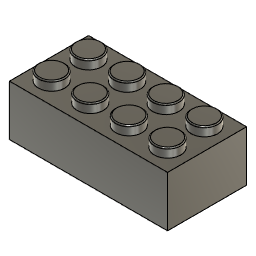
lago v2 (Autodesk Fusion 360 design; units mm, degrees)
Autodesk Fusion 360 part; units mm, degrees
note: some values were not read from the file. Set by a fixed rule: which face or edge a step refers to.
sketch "Sketch1" plane through (0, 0, 0) normal (0, 0, 1) x (1, 0, 0) in component "lago"
  line L0 (0, 0) -> (30, 0)
  line L1 (30, 0) -> (30, 15)
  line L2 (30, 15) -> (0, 15)
  line L3 (0, 15) -> (0, 0)
  constraint horizontal L0
  constraint vertical L1
  constraint horizontal L2
  constraint vertical L3
  constraint coincident L0.start L3.end
extrude "Extrude1" add sketch "Sketch1" along normal blind 9.6 in component "lago"
sketch "Sketch2" plane through (0, 0, 9.6) normal (0, 0, 1) x (-1, 0, 0) in component "lago"
  line L0 (0, -15) -> (0, 0)
  line L1 (0, 0) -> (-30, 0)
  line L2 (-30, 0) -> (-30, -15)
  line L3 (-30, -15) -> (0, -15)
  circle A0 centre (-3.9, -11.1) radius 2.5
  dimension "d3" = 5
  dimension "d4" = 3.9
  dimension "d5" = 3.9
  measures "d3" diameter of A0
  measures "d4" distance of L3 A0.centre
  measures "d5" distance of L0 A0.centre
extrude "Extrude2" add sketch "Sketch2" along normal blind 1.7 contours A0 in component "lago"
pattern_linear "R-Pattern1" count 4 spacing 7.3333 along (1, 0, 0) count 2 spacing 7 along (0, -1, 0) of "Extrude2" in component "lago"
shell "Shell1" thickness 1.3 removed faces 1 at (10, 5, 0) in component "lago"
sketch "Sketch3" plane through (0, 0, 8.3) normal (0, 0, -1) x (1, 0, 0) in component "lago"
  circle A0 centre (25.9, -4.1) radius 1.2
  circle A1 centre (18.5667, -4.1) radius 1.2
  circle A2 centre (11.2333, -4.1) radius 1.2
  circle A3 centre (3.9, -4.1) radius 1.2
  circle A4 centre (25.9, -11.1) radius 1.2
  circle A5 centre (18.5667, -11.1) radius 1.2
  circle A6 centre (11.2333, -11.1) radius 1.2
  circle A7 centre (3.9, -11.1) radius 1.2
  line L0 (1.3, -1.3) -> (1.3, -13.7)
  line L1 (1.3, -13.7) -> (28.7, -13.7)
  line L2 (28.7, -13.7) -> (28.7, -1.3)
  line L3 (28.7, -1.3) -> (1.3, -1.3)
  line L4 (11.2333, -4.1) -> (3.9, -11.1) construction
  circle A8 centre (7.5667, -7.6) radius 2.3581
  circle A9 centre (7.5667, -7.6) radius 3.3581
  dimension "d13" = 1
  constraint coincident A2.centre L4.start
  constraint coincident A7.centre L4.end
  constraint midpoint L4 A8.centre
extrude "Extrude3" add sketch "Sketch3" along normal blind 8 contours A9 in component "lago"
pattern_linear "R-Pattern2" count 3 spacing 7.5 along (1, 0, 0) of "Extrude3" in component "lago"
fillet "Fillet1" radius 0.2 8 edges at (28.2308, 12.004, 11.3) (28.2308, 5.004, 11.3) (20.8975, 5.004, 11.3) (20.8975, 12.004, 11.3) (13.5642, 5.004, 11.3) (13.5642, 12.004, 11.3) (6.2308, 12.004, 11.3) (6.2308, 5.004, 11.3) in component "lago"
fillet "Fillet2" radius 0.02 3 edges at (19.4358, 8.8143, 0.3) (11.9358, 8.8143, 0.3) (4.4358, 8.8143, 0.3) in component "lago"
fillet "Fillet3" radius 0.02 2 edges at (11.9358, 6.3857, 8.3) (4.4358, 6.3857, 8.3) in component "lago"
fillet "Fillet4" radius 0.2 1 edges at (19.4358, 6.3857, 8.3) in component "lago"
fillet "Fillet5" radius 0.2 13 faces at (10.5569, 7.883, 0.3) (10.9077, 7.2657, 0.3165) (10.908, 7.9344, 5.6267) (9.5276, 10.3275, 8.2868) (28.1489, 6.4846, 8.3) (9.5276, 10.3275, 8.2868) (18.408, 7.9344, 5.6267) (10.9077, 7.2657, 0.3165) (18.0656, 7.7658, 0.3) (24.1856, 10.7578, 8.2998) (25.9206, 7.7674, 2.9133) (10.9077, 7.2657, 0.3165) (25.5656, 7.7658, 0.3) in component "lago"
component "lago" placed x (1, 0, 0) y (0, 1, 0) z (0, 0, 1) at (0, 0, 0)
